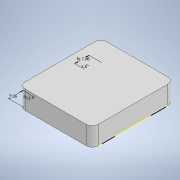
# Autodesk Inventor part: Bottom
Saved by Autodesk Inventor 2020 (Build 240168000, 168)
## iProperties
Created: 2021-08-22
Part Number: Bottom
Material: Generic
Document SubType Name: Modeling
Designer: nigel
Density: 1 g/cm^3
Appearance: Default
Author: nigel
Autodesk Inventor part; units mm, degrees
ref_plane "YZ Plane" through (0, 0, 0) normal (1, 0, 0) x (0, 1, 0)
ref_plane "XZ Plane" through (0, 0, 0) normal (0, 1, 0) x (-1, 0, 0)
ref_plane "XY Plane" through (0, 0, 0) normal (0, 0, 1) x (1, 0, 0)
sketch "Sketch1" plane through (0, 0, 0) normal (0, 1, 0) x (-1, 0, 0)
  line L0 (17, 19.1) -> (-17, 19.1)
  line L1 (-17, 19.1) -> (-17, -19.1)
  line L2 (-17, -19.1) -> (17, -19.1)
  line L3 (17, -19.1) -> (17, 19.1)
  line L4 (17, 19.1) -> (-17, -19.1) construction
  line L5 (-17, 19.1) -> (17, -19.1) construction
  line L6 (-18, 20.1) -> (18, 20.1)
  line L7 (18, 20.1) -> (18, -20.1)
  line L8 (18, -20.1) -> (-18, -20.1)
  line L9 (-18, -20.1) -> (-18, 20.1)
  line L10 (-18, 20.1) -> (18, -20.1) construction
  line L11 (18, 20.1) -> (-18, -20.1) construction
  point P0 (0, 0)
  point P1 (0, 0)
  point P2 (0, 0)
  dimension "d0" = 38.2
  dimension "d5" = 34
  dimension "d94" = 1
  dimension "d95" = 1
  constraints: 24 end point, 6 midpoint, 4 parallel, 2 horizontal, 2 perpendicular
  measures "d0" distance of L0.end L1.end
  measures "d5" distance of L1.end L2.end
  measures "d94" distance between parallel lines of L7 L3
  measures "d95" distance between parallel lines of L8 L2
extrude "Extrusion1" add sketch "Sketch1" along normal blind 9.14 contours L3 L2 L1 L0 | L6 L7 L8 L9
extrude "Extrusion14" cut sketch "Sketch1" along normal blind 0.94 contours L3 L2 L1 L0
sketch "Sketch15" plane through (0, 0.94, 0) normal (0, -1, 0) x (1, 0, 0)
  line L0 (-17, -19.1) -> (-17, 19.1) projected
  line L1 (17, 17.6) -> (-17, 17.6)
  line L2 (-17, 17.6) -> (-17, -17.6)
  line L3 (-17, -17.6) -> (17, -17.6)
  line L4 (17, -17.6) -> (17, 17.6)
  line L5 (17, 17.6) -> (-17, -17.6) construction
  line L6 (-17, 17.6) -> (17, -17.6) construction
  line L7 (17, -19.1) -> (-17, -19.1) projected
  point P0 (0, 0)
  dimension "d98" = 1.5
  constraints: 12 end point, 2 midpoint, 2 parallel, 1 horizontal, 1 perpendicular, 1 point on line
  measures "d98" distance between parallel lines of L3 L7
extrude "Extrusion15" cut sketch "Sketch15" against normal blind 3 from surface at 0.94
sketch "Sketch16" plane through (-17, 3, -17.6) normal (0, -1, 0) x (1, 0, 0)
  line L0 (31.5, 31.2) -> (2.5, 31.2)
  line L1 (2.5, 31.2) -> (2.5, 4)
  line L2 (2.5, 4) -> (31.5, 4)
  line L3 (31.5, 4) -> (31.5, 31.2)
  line L4 (31.5, 31.2) -> (2.5, 4) construction
  line L5 (2.5, 31.2) -> (31.5, 4) construction
  line L6 (34, -1.5) -> (0, -1.5) projected
  line L7 (0, -1.5) -> (0, 36.7) projected
  point P0 (17, 17.6)
  dimension "d101" = 5.5
  dimension "d102" = 2.5
  constraints: 12 end point, 2 midpoint, 2 parallel, 1 horizontal, 1 perpendicular
  measures "d101" distance between parallel lines of L6 L2
  measures "d102" distance between parallel lines of L7 L1
extrude "Extrusion17" cut sketch "Sketch16" against normal blind 3.5 from surface at 2.06
sketch "Sketch17" plane through (-17, 0.94, -17.6) normal (0, -1, 0) x (1, 0, 0)
  line L0 (29, 34.1) -> (8, 34.1)
  line L1 (8, 34.1) -> (8, 1.1)
  line L2 (8, 1.1) -> (29, 1.1)
  line L3 (29, 1.1) -> (29, 34.1)
  line L4 (29, 34.1) -> (8, 1.1) construction
  line L5 (8, 34.1) -> (29, 1.1) construction
  line L6 (34, 36.7) -> (34, -1.5) projected
  line L7 (0, -1.5) -> (0, 36.7) projected
  line L8 (34, 36.7) -> (34, 35.2) projected
  line L9 (34, -1.5) -> (0, -1.5) projected
  line L10 (34, 36.7) -> (0, -1.5) construction
  line L11 (34, -1.5) -> (0, 36.7) construction
  point P0 (18.5, 17.6)
  point P1 (18.5, 17.6)
  point P2 (17, 17.6)
  dimension "d105" = 33
  dimension "d106" = 5
  dimension "d107" = 8
  constraints: 16 end point, 4 midpoint, 2 parallel, 1 horizontal, 1 horizontal alignment, 1 perpendicular
  measures "d105" distance of L2.end L0.start
  measures "d106" distance between parallel lines of L6 L3
  measures "d107" distance between parallel lines of L7 L1
extrude "Extrusion18" cut sketch "Sketch17" against normal blind 7.2 from surface at 0
sketch "Sketch18" plane through (-17, 3, -17.6) normal (0, -1, 0) x (1, 0, 0)
  line L0 (31.5, 4) -> (31.5, 31.2) projected
  line L1 (34, 24.2) -> (31.5, 24.2)
  line L2 (31.5, 24.2) -> (31.5, 11)
  line L3 (31.5, 11) -> (34, 11)
  line L4 (34, 11) -> (34, 24.2)
  line L5 (34, 36.7) -> (34, -1.5) projected
  line L6 (0, 35.2) -> (34, 35.2) projected
  line L7 (34, 0) -> (0, 0) projected
  point P0 (17, 17.6)
  dimension "d112" = 11
  dimension "d113" = 11
  constraints: 8 end point, 2 parallel, 2 point on line, 1 horizontal, 1 perpendicular
  measures "d112" distance between parallel lines of L6 L1
  measures "d113" distance between parallel lines of L7 L3
extrude "Extrusion19" cut sketch "Sketch18" against normal blind 2.5 from surface at 2.06
fillet "Fillet7" radius 3 4 edges at (18, 4.57, 20.1) (18, 4.57, -20.1) (-18, 4.57, -20.1) (-18, 4.57, 20.1)
fillet "Fillet7" radius 0.5 4 edges at (17, 0.47, 19.1) (17, 0.47, -19.1) (-17, 0.47, -19.1) (-17, 0.47, 19.1)
sketch "Sketch19" plane through (0, 0, 0) normal (0, -1, 0) x (1, 0, 0)
  line L0 (-18, -17.1) -> (-18, 17.1) projected
  line L1 (-18, 3.5) -> (-9, 3.5)
  line L2 (-9, 3.5) -> (-9, -4.7)
  line L3 (-9, -4.7) -> (-18, -4.7)
  line L4 (-18, -4.7) -> (-18, 3.5)
  line L5 (-9, -13.6) -> (-9, 13.6) projected
  line L6 (-16.5, 19.1) -> (16.5, 19.1) projected
  point P0 (0, 0)
  dimension "d118" = 8.2
  dimension "d120" = 23.8
  constraints: 8 end point, 2 parallel, 1 collinear, 1 horizontal, 1 perpendicular, 1 point on line
  measures "d118" distance of L1.end L2.end
  measures "d120" distance between parallel lines of L6 L3
extrude "Extrusion20" cut sketch "Sketch19" against normal blind 4
sketch "Sketch22" plane through (0, 0, 0) normal (0, -1, 0) x (1, 0, 0)
  line L0 (17, 6.6) -> (17, 17.6) projected
  line L1 (18, 17.1) -> (18, -17.1) projected
  line L2 (17, 15.4691) -> (18, 15.4691)
  line L3 (18, 15.4691) -> (18, 9.1584)
  line L4 (18, 9.1584) -> (17, 9.1584)
  line L5 (17, 9.1584) -> (17, 15.4691)
  line L6 (17, -17.6) -> (17, -6.6) projected
  line L7 (17, -15.963) -> (18, -15.963)
  line L8 (18, -15.963) -> (18, -8.6814)
  line L9 (18, -8.6814) -> (17, -8.6814)
  line L10 (17, -8.6814) -> (17, -15.963)
  line L11 (-18, -17.1) -> (-18, 17.1) projected
  line L12 (-17, 15.8937) -> (-18, 15.8937)
  line L13 (-18, 15.8937) -> (-18, 10.7863)
  line L14 (-18, 10.7863) -> (-17, 10.7863)
  line L15 (-17, 10.7863) -> (-17, 15.8937)
  line L16 (-17, 15.8937) -> (-18, 10.7863) construction
  line L17 (-18, 15.8937) -> (-17, 10.7863) construction
  line L18 (-17, -11.5535) -> (-18, -11.5535)
  line L19 (-18, -11.5535) -> (-18, -15.1265)
  line L20 (-18, -15.1265) -> (-17, -15.1265)
  line L21 (-17, -15.1265) -> (-17, -11.5535)
  line L22 (-17, -11.5535) -> (-18, -15.1265) construction
  line L23 (-18, -11.5535) -> (-17, -15.1265) construction
  line L24 (-17, -18.6) -> (-17, -4.7) projected
  line L25 (-17, 3.5) -> (-17, 18.6) projected
  line L26 (-17, 14.64) -> (-18, 14.64) construction
  line L27 (-18, 14.64) -> (-18, 12.04) construction
  line L28 (-18, 12.04) -> (-17, 12.04) construction
  line L29 (-17, 12.04) -> (-17, 14.64) construction
  line L30 (-17, 14.64) -> (-18, 12.04) construction
  line L31 (-18, 14.64) -> (-17, 12.04) construction
  line L32 (-17, -12.04) -> (-18, -12.04) construction
  line L33 (-18, -12.04) -> (-18, -14.64) construction
  line L34 (-18, -14.64) -> (-17, -14.64) construction
  line L35 (-17, -14.64) -> (-17, -12.04) construction
  line L36 (-17, -12.04) -> (-18, -14.64) construction
  line L37 (-18, -12.04) -> (-17, -14.64) construction
  line L38 (-16.5, 19.1) -> (16.5, 19.1) construction
  line L39 (16.5, -19.1) -> (-16.5, -19.1) construction
  point P0 (0, 0)
  point P1 (-17.5, 13.34)
  point P2 (-17.5, -13.34)
  dimension "d123" = 2.6
  dimension "d124" = 2.6
  dimension "d125" = 7.06
  dimension "d126" = 7.06
  constraints: 64 end point, 12 parallel, 8 midpoint, 8 point on line, 6 horizontal, 6 perpendicular, 2 collinear
  measures "d123" distance between parallel lines of L32 L34
  measures "d124" distance between parallel lines of L28 L26
  measures "d125" distance between parallel lines of L38 L28
  measures "d126" distance between parallel lines of L39 L32
equation "\"d6\" = PCB_thickness + electronics_thickness + case_thickness"
equation "\"PCB_thickness\" = 0.94"
equation "\"case_thickness\" = 1"
equation "\"electronics_thickness\" = 7.2"
equation "\"usb_height\" = 4"
body "Solid1"
